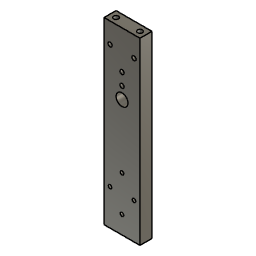
hub_mount (Autodesk Fusion 360 design; units mm, degrees)
Autodesk Fusion 360 part; units mm, degrees
sketch "Sketch1" plane through (0, 0, 0) normal (0, 0, 1) x (1, 0, 0)
  line L0 (15, 5) -> (-15, 5)
  line L1 (-15, 5) -> (-15, -5)
  line L2 (-15, -5) -> (15, -5)
  line L3 (15, -5) -> (15, 5)
  line L4 (15, 5) -> (-15, -5) construction
  line L5 (-15, 5) -> (15, -5) construction
  dimension "d1" = 30
  dimension "d2" = 10
  constraint horizontal L0
  constraint perpendicular L0 L1
  constraint parallel L0 L2
  constraint parallel L1 L3
  constraint coincident L4 origin
  constraint coincident L5 origin
  measures "d1" distance of L1.end L2.end
  measures "d2" distance of L0.end L1.end
extrude "Extrude1" add sketch "Sketch1" along normal blind 150
sketch "Sketch2" plane through (0, -5, 0) normal (0, -1, 0) x (1, 0, 0)
  line L0 (-15, 0) -> (15, 0)
  line L1 (15, 0) -> (15, 150)
  line L2 (15, 150) -> (-15, 150)
  line L3 (-15, 150) -> (-15, 0)
  circle A0 centre (0, 118) radius 1.75
  line L4 (0, 150) -> (0, 118)
  circle A1 centre (-10, 133) radius 1.75
  circle A2 centre (10, 133) radius 1.75
  dimension "d5" = 3.5
  dimension "d6" = 32
  dimension "d7" = 3.5
  dimension "d8" = 3.5
  dimension "d9" = 10
  dimension "d10" = 10
  dimension "d11" = 15
  dimension "d12" = 15
  constraint midpoint L2 L4.start
  constraint perpendicular L2 L4
  constraint coincident A0.centre L4.end
  measures "d5" diameter of A0
  measures "d6" distance of L2 A0.centre
  measures "d7" diameter of A1
  measures "d8" diameter of A2
  measures "d9" distance of L4 A1.centre
  measures "d10" distance of L4 A2.centre
  measures "d11" vertical distance of A0.centre A1.centre
  measures "d12" vertical distance of A0.centre A2.centre
extrude "Extrude2" cut sketch "Sketch2" against normal blind 10 contours A0 | A1 | A2
sketch "Sketch3" plane through (0, 0, 150) normal (0, 0, 1) x (-1, 0, 0)
  line L0 (-15, 5) -> (-15, -5)
  line L1 (-15, -5) -> (15, -5)
  line L2 (15, -5) -> (15, 5)
  line L3 (15, 5) -> (-15, 5)
  circle A0 centre (10, 0) radius 2.05
  circle A1 centre (-10, 0) radius 2.05
  dimension "d15" = 4.1
  dimension "d17" = 10
  dimension "d18" = 10
  constraint equal A0 A1
  constraint horizontal origin A0.centre
  constraint horizontal origin A1.centre
  measures "d15" diameter of A0
  measures "d17" distance of origin A0.centre
  measures "d18" distance of origin A1.centre
extrude "Extrude3" cut sketch "Sketch3" against normal blind 12 contours A0 | A1
sketch "Sketch4" plane through (0, -5, 0) normal (0, -1, 0) x (1, 0, 0)
  circle A0 centre (-10, 133) radius 1.75
  circle A1 centre (10, 133) radius 1.75
  circle A2 centre (0, 118) radius 1.75
  line L0 (-15, 0) -> (15, 0)
  line L1 (15, 0) -> (15, 150)
  line L2 (15, 150) -> (-15, 150)
  line L3 (-15, 150) -> (-15, 0)
  line L4 (0, 0) -> (0, 6)
  circle A3 centre (0, 15) radius 1.5
  circle A4 centre (-10, 30) radius 1.5
  circle A5 centre (10, 30) radius 1.5
  circle A6 centre (0, 45) radius 1.5
  dimension "d21" = 3
  dimension "d22" = 15
  dimension "d23" = 3
  dimension "d24" = 10
  dimension "d25" = 30
  dimension "d26" = 3
  dimension "d27" = 45
  constraint coincident L4.start origin
  constraint perpendicular L0 L4
  constraint coincident L4 A3.centre
  constraint symmetric L4 A4 A5
  constraint coincident L4 A6.centre
  measures "d21" diameter of A3
  measures "d22" distance of L0 A3.centre
  measures "d23" diameter of A4
  measures "d24" horizontal distance of L4.start A4.centre
  measures "d25" vertical distance of L4.start A4.centre
  measures "d26" diameter of A6
  measures "d27" distance of L0 A6.centre
extrude "Extrude4" cut sketch "Sketch4" against normal blind 10 contours A3 | A4 | A5 | A6
sketch "Sketch5" plane through (0, -5, 0) normal (0, -1, 0) x (1, 0, 0)
  circle A0 centre (0, 45) radius 1.5
  circle A1 centre (10, 30) radius 1.5
  circle A2 centre (-10, 30) radius 1.5
  circle A3 centre (0, 15) radius 1.5
  circle A4 centre (-10, 133) radius 1.75
  circle A5 centre (10, 133) radius 1.75
  circle A6 centre (0, 118) radius 1.75
  line L0 (-15, 0) -> (15, 0)
  line L1 (15, 0) -> (15, 150)
  line L2 (15, 150) -> (-15, 150)
  line L3 (-15, 150) -> (-15, 0)
  circle A7 centre (0, 108) radius 1.75
  dimension "d30" = 3.5
  dimension "d31" = 10
  measures "d30" diameter of A7
  measures "d31" distance of A6.centre A7.centre
extrude "Extrude5" cut sketch "Sketch5" against normal blind 10 contours A7
sketch "Sketch6" plane through (0, -5, 0) normal (0, -1, 0) x (1, 0, 0)
  circle A0 centre (0, 108) radius 1.75
  circle A1 centre (0, 45) radius 1.5
  circle A2 centre (10, 30) radius 1.5
  circle A3 centre (-10, 30) radius 1.5
  circle A4 centre (0, 15) radius 1.5
  circle A5 centre (-10, 133) radius 1.75
  circle A6 centre (10, 133) radius 1.75
  circle A7 centre (0, 118) radius 1.75
  line L0 (-15, 0) -> (15, 0)
  line L1 (15, 0) -> (15, 150)
  line L2 (15, 150) -> (-15, 150)
  line L3 (-15, 150) -> (-15, 0)
  circle A8 centre (0, 98) radius 5
  dimension "d34" = 10
  dimension "d35" = 10
  measures "d34" diameter of A8
  measures "d35" distance of A0.centre A8.centre
extrude "Extrude6" cut sketch "Sketch6" against normal blind 10 contours A8
